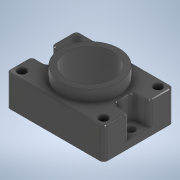
# Autodesk Inventor part: rpiCamM12Mount
Saved by Autodesk Inventor 2020 (Build 240168000, 168)
## iProperties
Created: 2019-08-05
Part Number: rpiCamM12Mount
Material: Generic
Document SubType Name: Modeling
Designer: n10208577
Density: 1 g/cm^3
Appearance: Default
Author: n10208577
Autodesk Inventor part; units mm, degrees
ref_plane "YZ Plane" through (0, 0, 0) normal (1, 0, 0) x (0, 1, 0)
ref_plane "XZ Plane" through (0, 0, 0) normal (0, 1, 0) x (-1, 0, 0)
ref_plane "XY Plane" through (0, 0, 0) normal (0, 0, 1) x (1, 0, 0)
sketch "Sketch1" plane through (0, 0, 0) normal (0, 1, 0) x (-1, 0, 0)
  circle A0 centre (0, 0) radius 1.1
  line L0 (0, 0) -> (-21, 0)
  circle A1 centre (-21, 0) radius 1.1
  line L1 (0, 0) -> (2, 0)
  line L2 (-21, 0) -> (-23, 0)
  circle A2 centre (-10.5, 0) radius 6
  line L3 (0, 0) -> (0, -7)
  line L4 (0, 0) -> (0, 7)
  line L5 (-21, 0) -> (-21, -7)
  line L6 (-21, 0) -> (-21, 7)
  circle A3 centre (0, -7) radius 1.1
  circle A4 centre (0, 7) radius 1.1
  circle A5 centre (-21, 7) radius 1.1
  circle A6 centre (-21, -7) radius 1.1
  line L7 (2, 0) -> (2, 9)
  line L8 (2, 9) -> (-23, 9)
  line L9 (-23, 9) -> (-23, -9)
  line L10 (-23, -9) -> (2, -9)
  line L11 (2, -9) -> (2, 9)
  dimension "d0" = 2.2
  dimension "d1" = 21
  dimension "d2" = 2.2
  dimension "d3" = 2
  dimension "d4" = 2
  dimension "d5" = 12
  dimension "d6" = 7
  dimension "d7" = 7
  dimension "d8" = 7
  dimension "d9" = 7
  dimension "d10" = 2.2
  dimension "d11" = 2.2
  dimension "d12" = 2.2
  dimension "d13" = 2.2
  dimension "d14" = 9
  dimension "d15" = 25
  dimension "d16" = 18
  constraints: 24 end point, 7 centre point, 6 coincident, 5 vertical, 4 horizontal, 2 parallel, 1 midpoint, 1 perpendicular
  measures "d0" diameter of A0
  measures "d1" distance of L0.start L0.end
  measures "d2" diameter of A1
  measures "d3" distance of L0.start L1.end
  measures "d4" distance of L2.start L2.end
  measures "d5" diameter of A2
  measures "d6" distance of L0.start L3.end
  measures "d7" distance of L0.start L4.end
  measures "d8" distance of L2.start L5.end
  measures "d9" distance of L2.start L6.end
  measures "d10" diameter of A3
  measures "d11" diameter of A4
  measures "d12" diameter of A5
  measures "d13" diameter of A6
  measures "d14" distance of L1.end L7.end
  measures "d15" distance of L10.end L9.end
  measures "d16" distance of L9.end L8.end
extrude "Extrusion1" add sketch "Sketch1" along normal blind 2 contours L1 L11 L10 L9 L2 A1 L0 A2 A0 | A0 L0 A2 A1 L2 L9 L8 L7 L1
sketch "Sketch2" plane through (0, 2, 0) normal (0, 1, 0) x (1, 0, 0)
  line L0 (-2, -9) -> (23, -9) projected
  line L1 (23, -9) -> (23, 9) projected
  line L2 (23, 9) -> (-2, 9) projected
  line L3 (-2, 9) -> (-2, -9) projected
  circle A0 centre (21, 7) radius 1.1 projected
  circle A1 centre (0, 7) radius 1.1 projected
  circle A2 centre (0, -7) radius 1.1 projected
  circle A3 centre (0, 0) radius 1.1 projected
  circle A4 centre (10.5, 0) radius 6 projected
  circle A5 centre (21, -7) radius 1.1 projected
  circle A6 centre (21, 0) radius 1.1 projected
  line L4 (0, 0) -> (0, -2.5)
  circle A7 centre (0, 0) radius 1.1 projected
  line L5 (0, 0) -> (0, 2.5)
  line L6 (0, 0) -> (2, 0)
  line L7 (0, -2.5) -> (2, -2.5)
  line L8 (2, -2.5) -> (2, 0)
  line L9 (2, 2.5) -> (0, 2.5)
  line L10 (0, 2.5) -> (-2, 2.5)
  line L11 (-2, 9) -> (-2, -9) projected
  line L12 (0, -2.5) -> (-2, -2.5)
  line L13 (21, 0) -> (19, 0)
  line L14 (19, 0) -> (19, -2.5)
  line L15 (19, -2.5) -> (23, -2.5)
  line L16 (19, 0) -> (19, 2.5)
  line L17 (19, 2.5) -> (23, 2.5)
  line L18 (23, -9) -> (23, 9) projected
  line L19 (2, 2.5) -> (2, 0)
  dimension "d19" = 2.5
  dimension "d20" = 2.5
  dimension "d21" = 2
  dimension "d22" = 2
  dimension "d23" = 2
  dimension "d24" = 2.5
  dimension "d25" = 2.5
  constraints: 28 end point, 10 point on line, 2 horizontal, 2 perpendicular, 2 vertical, 1 parallel
  measures "d19" distance of L4.start L4.end
  measures "d20" distance of L5.start L5.end
  measures "d21" distance of L5.start L6.end
  measures "d22" distance of L4.end L7.end
  measures "d23" distance of L13.start L13.end
  measures "d24" distance of L13.end L14.end
  measures "d25" distance of L13.end L16.end
extrude "Extrusion2" add sketch "Sketch2" along normal blind 6 contours L3 L12 L7 L8 L19 L9 L10 L2 L1 L17 L16 L14 L15 L0
fillet "Fillet1" radius 1 12 edges at (2, 5, 2.5) (2, 5, -2.5) (19, 5, 2.5) (19, 5, -2.5) (23, 5, -2.5) (23, 4, 9) (23, 5, 2.5) (-2, 4, 9) (-2, 5, 2.5) (-2, 5, -2.5) (-2, 4, -9) (23, 4, -9)
chamfer "Chamfer1" distance 0.25 angle 45 24 edges at (10.5, 8, 9) (22.7071, 8, 8.7071) (23, 8, 5.75) (22.7071, 8, 2.7929) (21, 8, 2.5) (19.2929, 8, 2.2071) (19, 8, 0) (19.2929, 8, -2.2071) (21, 8, -2.5) (22.7071, 8, -2.7929) (23, 8, -5.75) (22.7071, 8, -8.7071) (10.5, 8, -9) (-1.7071, 8, -8.7071) (-2, 8, -5.75) (-2, 8, 5.75) (-1.7071, 8, -2.7929) (0, 8, -2.5) (1.7071, 8, -2.2071) (2, 8, 0) (1.7071, 8, 2.2071) (0, 8, 2.5) (-1.7071, 8, 2.7929) (-1.7071, 8, 8.7071)
sketch "Sketch3" plane through (0, 8, 0) normal (0, 1, 0) x (1, 0, 0)
  circle A0 centre (10.5, 0) radius 6 projected
  circle A1 centre (10.5, 0) radius 7.5
  point P0 (0, 0)
  dimension "d32" = 15
  constraints: 1 centre point, 1 coincident
  measures "d32" diameter of A1
extrude "Extrusion3" add sketch "Sketch3" along normal blind 3
body "Solid1"
